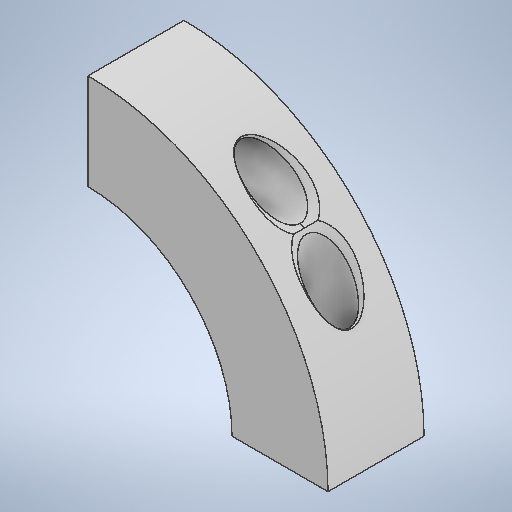
# Autodesk Inventor part: RT_FRM_MC_013_R100_Door_Roundover
Saved by Autodesk Inventor 2025.3 (Build 293356000, 356)
## iProperties
Created: 2026-06-06
Part Number: RT_FRM_MC_013_R100_Door_Roundover
Material: Generic
Document SubType Name: Modeling
Designer: louis
Density: 1 g/cm^3
Appearance: Default
Author: louis
Autodesk Inventor part; units mm, degrees
ref_plane "YZ Plane" through (0, 0, 0) normal (1, 0, 0) x (0, 1, 0)
ref_plane "XZ Plane" through (0, 0, 0) normal (0, 1, 0) x (-1, 0, 0)
ref_plane "XY Plane" through (0, 0, 0) normal (0, 0, 1) x (1, 0, 0)
sketch "Sketch1" plane through (0, 0, 0) normal (0, 0, 1) x (1, 0, 0)
  arc A0 (100, 0) -> (0, 100) centre (0, 0) ccw
  arc A1 (60, 0) -> (0, 60) centre (0, 0) ccw
  line L0 (0, 60) -> (0, 100)
  line L1 (60, 0) -> (100, 0)
  line L2 (0, 0) -> (0, 60) construction
  line L3 (60, 0) -> (0, 0) construction
  dimension "d5" = 200
  dimension "d6" = 120
  constraints: 8 end point, 4 point on circle, 2 centre point, 2 coincident, 1 collinear, 1 horizontal, 1 perpendicular, 1 vertical
  measures "d5" diameter of A0
  measures "d6" diameter of A1
extrude "Extrusion1" add sketch "Sketch1" along normal mid plane 40
ref_plane "Work Plane1" through (60, 5, 20) normal (0, -1, 0) x (1, 0, 0)
sketch "Sketch2" plane through (60, 5, 20) normal (0, -1, 0) x (1, 0, 0)
  line L0 (0, -40) -> (0, 0) construction
  line L1 (40, 0) -> (-60, 0) construction
  line L2 (0, -40) -> (40, 0) construction
  point P0 (-60, -20)
  point P1 (20, -20)
  constraints: 2 end point, 1 midpoint
hole "Hole1" at (80, 5, 0) direction (0, -1, 0) diameter 10 end through all start extended yes counterbore diameter 18.01 counterbore depth 0.5
chamfer "Chamfer1" distance 2 angle 45 1 edges at (70.995, 70.4252, -0.0047)
ref_plane "Work Plane2" through (0, 0, 20) normal (0.7071068, -0.7071068, 0) x (0, 0, 1)
mirror "Mirror1" about plane through (0, 0, 20) normal (0.7071068, -0.7071068, 0) of "Hole1", "Chamfer1"
body "Solid1"
